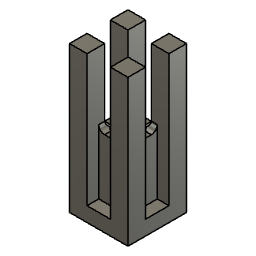
Pillar 2cm_ (Autodesk Fusion 360 design; units mm, degrees)
Autodesk Fusion 360 part; units mm, degrees
sketch "Esquisse1" plane through (0, 0, 0) normal (0, 1, 0) x (1, 0, 0)
  line L0 (-20, 20) -> (0, 20)
  line L1 (0, 20) -> (0, 0)
  line L2 (0, 0) -> (-20, 0)
  line L3 (-20, 0) -> (-20, 20)
  line L4 (-20, 14) -> (-14, 14)
  line L5 (-14, 20) -> (-14, 14)
  circle A0 centre (-10, 10) radius 1.75
  line L6 (-20, 6) -> (-14, 6)
  line L7 (-14, 0) -> (-14, 6)
  line L8 (-6, 0) -> (-6, 6)
  line L9 (0, 6) -> (-6, 6)
  line L10 (0, 14) -> (-6, 14)
  line L11 (-6, 20) -> (-6, 14)
  line L12 (-16, 14) -> (-16, 6)
  line L13 (-14, 15.9988) -> (-6, 15.9988)
  line L14 (-4, 14) -> (-4, 6)
  line L15 (-6, 4) -> (-14, 4)
  line L16 (-14, 14) -> (-6, 14)
  line L17 (-6, 14) -> (-6, 6)
  line L18 (-6, 6) -> (-14, 6)
  line L19 (-14, 6) -> (-14, 14)
  line L20 (-11.6634, 12.7724) -> (-13.2327, 9.9456)
  line L21 (-13.2327, 9.9456) -> (-11.5693, 7.1732)
  line L22 (-11.5693, 7.1732) -> (-8.3366, 7.2276)
  line L23 (-8.3366, 7.2276) -> (-6.7673, 10.0544)
  line L24 (-6.7673, 10.0544) -> (-8.4307, 12.8268)
  line L25 (-8.4307, 12.8268) -> (-11.6634, 12.7724)
  point P0 (-10, 10)
  dimension "d1" = 20
  dimension "d2" = 20
  dimension "d3" = 6
  dimension "d4" = 6
  dimension "d5" = 3.5
  dimension "d6" = 10
  dimension "d7" = 10
  dimension "d9" = 360
  dimension "d10" = 2
  dimension "d11" = 2
  dimension "d12" = 2
  dimension "d22" = 8
  dimension "d23" = 5.6
  constraint horizontal L0
  constraint vertical L1
  constraint horizontal L2
  constraint vertical L3
  constraint coincident L1.end L2.start
  constraint coincident L3 L4.start
  constraint perpendicular L3 L4
  constraint coincident L0 L5.start
  constraint perpendicular L4 L5
  constraint coincident L4 L12.start
  constraint coincident L6 L12.end
  constraint perpendicular L6 L12
  constraint coincident L5 L13.start
  constraint coincident L11 L13.end
  constraint perpendicular L11 L13
  constraint coincident L10 L14.start
  constraint coincident L9 L14.end
  constraint perpendicular L9 L14
  constraint coincident L8 L15.start
  constraint coincident L7 L15.end
  constraint perpendicular L7 L15
  constraint horizontal L16
  constraint vertical L17
  constraint horizontal L18
  constraint vertical L19
  constraint coincident P0 A0.centre
  measures "d1" distance of L1.end L2.end
  measures "d2" distance of L0.end L1.end
  measures "d3" distance of L4.end L5.start
  measures "d4" distance of L4.start L4.end
  measures "d5" diameter of A0
  measures "d6" distance of L0 P0
  measures "d7" distance of L3 P0
  measures "d10" distance of L12 L19
  measures "d11" distance of L14 L17
  measures "d12" distance of L15 L18
  measures "d22" distance of L5 L11
  measures "d23" distance of L22 L25
extrude "Extrusion2" add sketch "Esquisse1" against normal blind 5 contours L0 L3 L4 L5 | L0 L5 L11 L13 | L3 L4 L6 L12 | L0 L1 L10 L11 | L5 L11 L13 L16 | L2 L3 L6 L7 | L4 L6 L12 L19 | L16 L17 L18 L19 | L1 L9 L10 L14 | L9 L10 L14 L17 | L7 L8 L15 L18 | L2 L7 L8 L15 | L1 L2 L8 L9 | L20 L21 L22 L23 L24 L25
extrude "Extrusion4" add sketch "Esquisse1" along normal blind 20 contours L0 L3 L4 L5 | L0 L1 L10 L11 | L5 L11 L13 L16 | L2 L3 L6 L7 | L4 L6 L12 L19 | L9 L10 L14 L17 | L7 L8 L15 L18 | L1 L2 L8 L9
sketch "Esquisse3" plane through (0, 20, 0) normal (0, 1, 0) x (-1, 0, 0)
  line L0 (6, -6) -> (14, -6)
  line L1 (14, -6) -> (14, -14)
  line L2 (14, -14) -> (6, -14)
  line L3 (6, -14) -> (6, -6)
  line L4 (0, -6) -> (4, -6)
  line L5 (4, -6) -> (4, -14)
  line L6 (4, -14) -> (0, -14)
  line L7 (0, -14) -> (0, -20)
  line L8 (0, -20) -> (6, -20)
  line L9 (6, -20) -> (6, -15.9988)
  line L10 (6, -15.9988) -> (14, -15.9988)
  line L11 (14, -15.9988) -> (14, -20)
  line L12 (14, -20) -> (20, -20)
  line L13 (20, -20) -> (20, -14)
  line L14 (20, -14) -> (16, -14)
  line L15 (16, -14) -> (16, -6)
  line L16 (16, -6) -> (20, -6)
  line L17 (20, -6) -> (20, 0)
  line L18 (20, 0) -> (14, 0)
  line L19 (14, 0) -> (14, -4)
  line L20 (14, -4) -> (6, -4)
  line L21 (6, -4) -> (6, 0)
  line L22 (6, 0) -> (0, 0)
  line L23 (0, 0) -> (0, -6)
  line L24 (20, -20) -> (14, -20)
  line L25 (14, -20) -> (14, -14)
  line L26 (14, -14) -> (20, -14)
  line L27 (20, -14) -> (20, -20)
  line L28 (0, -20) -> (6, -20)
  line L29 (6, -20) -> (6, -14)
  line L30 (6, -14) -> (0, -14)
  line L31 (0, -14) -> (0, -20)
  line L32 (0, -6) -> (6, -6)
  line L33 (6, -6) -> (6, 0)
  line L34 (6, 0) -> (0, 0)
  line L35 (0, 0) -> (0, -6)
  line L36 (14, -6) -> (20, -6)
  line L37 (20, -6) -> (20, 0)
  line L38 (20, 0) -> (14, 0)
  line L39 (14, 0) -> (14, -6)
  constraint horizontal L24
  constraint vertical L25
  constraint horizontal L26
  constraint vertical L27
  constraint coincident L1.end L2.start
  constraint coincident L12.end L13.start
  constraint horizontal L28
  constraint vertical L29
  constraint horizontal L30
  constraint vertical L31
  constraint coincident L2.end L3.start
  constraint coincident L7.end L8.start
  constraint horizontal L32
  constraint vertical L33
  constraint horizontal L34
  constraint vertical L35
  constraint coincident L21.end L22.start
  constraint coincident L4.start L23.end
  constraint horizontal L36
  constraint vertical L37
  constraint horizontal L38
  constraint vertical L39
  constraint coincident L17.end L18.start
  constraint coincident L0.end L1.start
extrude "Extrusion5" add sketch "Esquisse3" along normal blind 25 contours L4 L21 L22 L23 L32 L33 L34 L35 | L16 L17 L18 L19 L36 L37 L38 L39 | L6 L7 L8 L9 L28 L29 L30 L31 | L11 L12 L13 L14 L24 L25 L26 L27
extrude "Extrusion7" cut sketch "Esquisse1" against normal blind 3 contours L20 L21 L22 L23 L24 L25
extrude "Extrusion8" add 1 faces at (-12.934, 0, -7.7063) along direction (0, 1, 0) blind 1
fillet "Congé2" radius 3 4 edges at (-14, 10.5, -6) (-14, 10.5, -14) (-6, 10.5, -6) (-6, 10.5, -14)
fillet "Congé3" radius 2 8 edges at (-15, 20, -14) (-15, 20, -6) (-5, 20, -14) (-5, 20, -6) (-14, 20, -14.9994) (-6, 20, -14.9994) (-14, 20, -5) (-6, 20, -5)
